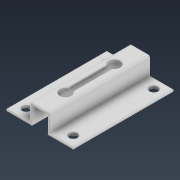
# Autodesk Inventor part: part1pasador
Saved by Autodesk Inventor 2021.2 (Build 252289000, 289)
## iProperties
Created: 2026-09-01
Part Number: part1pasador
Material: Generic
Document SubType Name: Modeling
Designer: Tecnica
Density: 1 g/cm^3
Appearance: Default
Author: Tecnica
Autodesk Inventor part; units mm, degrees
ref_plane "YZ Plane" through (0, 0, 0) normal (1, 0, 0) x (0, 1, 0)
ref_plane "XZ Plane" through (0, 0, 0) normal (0, 1, 0) x (-1, 0, 0)
ref_plane "XY Plane" through (0, 0, 0) normal (0, 0, 1) x (1, 0, 0)
sketch "Sketch1" plane through (0, 0, 0) normal (0, 1, 0) x (-1, 0, 0)
  line L0 (-20, 30) -> (20, 30)
  line L1 (20, 30) -> (20, -30)
  line L2 (20, -30) -> (-20, -30)
  line L3 (-20, -30) -> (-20, 30)
  line L4 (-20, 30) -> (20, -30) construction
  line L5 (20, 30) -> (-20, -30) construction
  point P0 (0, 0)
  dimension "d0" = 40
  dimension "d1" = 60
  constraints: 12 end point, 2 midpoint, 2 parallel, 1 horizontal, 1 perpendicular
  measures "d0" distance of L1.end L2.end
  measures "d1" distance of L0.end L1.end
extrude "Extrusion1" add sketch "Sketch1" along normal blind 12
sketch "Sketch2" plane through (-20, 0, 30) normal (0, 0, 1) x (1, 0, 0)
  line L0 (0, 0) -> (0, 12) projected
  line L1 (0, 0) -> (0, 1.45)
  line L2 (0, 1.45) -> (14, 1.45)
  line L3 (14, 1.45) -> (14, 12)
  line L4 (40, 12) -> (0, 12) projected
  line L5 (14, 12) -> (26, 12)
  line L6 (26, 12) -> (26, 1.45)
  line L7 (26, 1.45) -> (40, 1.45)
  line L8 (40, 0) -> (40, 12) projected
  line L9 (0, 12) -> (14, 12)
  line L10 (14, 12) -> (14, 1.45)
  line L11 (14, 1.45) -> (0, 1.45)
  line L12 (0, 1.45) -> (0, 12)
  line L13 (26, 1.45) -> (40, 1.45)
  line L14 (40, 1.45) -> (40, 12)
  line L15 (40, 12) -> (26, 12)
  line L16 (26, 12) -> (26, 1.45)
  line L17 (14, 1.45) -> (15.45, 1.45)
  line L18 (15.45, 1.45) -> (15.45, 12)
  line L19 (14, 12) -> (14, 10.55)
  line L20 (14, 10.55) -> (26, 10.55)
  line L21 (26, 12) -> (24.55, 12)
  line L22 (24.55, 12) -> (24.55, 1.45)
  line L23 (15.45, 10.55) -> (24.55, 10.55)
  line L24 (24.55, 10.55) -> (24.55, 0)
  line L25 (24.55, 0) -> (15.45, 0)
  line L26 (15.45, 0) -> (15.45, 10.55)
  point P0 (20, 0)
  point P1 (24.55, 1.45)
  point P2 (24.55, 10.55)
  point P3 (15.45, 1.45)
  dimension "d4" = 1.45
  dimension "d5" = 14
  dimension "d6" = 12
  dimension "d10" = 1.45
  dimension "d11" = 1.45
  dimension "d12" = 1.45
  constraints: 48 end point, 12 point on line, 10 perpendicular, 6 parallel, 4 horizontal
  measures "d4" distance of L0.start L1.end
  measures "d5" distance of L1.end L2.end
  measures "d6" distance of L3.end L5.end
  measures "d10" distance of L2.end L17.end
  measures "d11" distance of L9.end L19.end
  measures "d12" distance of L15.end L21.end
extrude "Extrusion2" cut sketch "Sketch2" against normal up to surface (60 mm away) contours L0 L4 L3 L2 | L18 L20 L22 L24 L25 L26 | L4 L8 L7 L6
fillet "Fillet1" radius 0.5 6 edges at (-20, 1.45, 0) (20, 1.45, 0) (-20, 0, 0) (20, 0, 0) (-4.55, 0, 0) (4.55, 0, 0)
fillet "Fillet1" radius 0.6 2 edges at (4.55, 10.55, 0) (-4.55, 10.55, 0)
fillet "Fillet1" radius 1.1 2 edges at (6, 12, 0) (-6, 12, 0)
sketch "Sketch3" plane through (-6, 1.45, 30) normal (0, 1, 0) x (1, 0, 0)
  line L0 (-14, 60) -> (-14, 0) projected
  line L1 (26, 0) -> (26, 60) projected
  line L2 (-14, 60) -> (26, 60)
  line L3 (26, 60) -> (26, 0)
  line L4 (26, 0) -> (-14, 0)
  line L5 (-14, 0) -> (-14, 60)
  line L6 (-14, 60) -> (-8, 60)
  line L7 (-8, 60) -> (-8, 54)
  line L8 (-8, 54) -> (-14, 54)
  line L9 (-14, 54) -> (-14, 60)
  circle A0 centre (-8, 54) radius 2.5
  line L10 (26, 60) -> (20, 60)
  line L11 (20, 60) -> (20, 54)
  line L12 (20, 54) -> (26, 54)
  line L13 (26, 54) -> (26, 60)
  circle A1 centre (20, 54) radius 2.5
  line L14 (26, 0) -> (25.5, 0) projected
  line L15 (26, 0) -> (20, 0)
  line L16 (20, 0) -> (20, 6)
  line L17 (20, 6) -> (26, 6)
  line L18 (26, 6) -> (26, 0)
  line L19 (-14, 0) -> (-8, 0)
  line L20 (-8, 0) -> (-8, 6)
  line L21 (-8, 6) -> (-14, 6)
  line L22 (-14, 6) -> (-14, 0)
  circle A2 centre (-8, 6) radius 2.5
  circle A3 centre (20, 6) radius 2.5
  point P0 (6, 30)
  dimension "d15" = 6
  dimension "d16" = 6
  dimension "d17" = 5
  dimension "d18" = 6
  dimension "d19" = 6
  dimension "d20" = 5
  dimension "d21" = 6
  dimension "d22" = 6
  dimension "d23" = 5
  dimension "d24" = 5
  dimension "d25" = 6
  dimension "d26" = 6
  constraints: 40 end point, 10 parallel, 5 horizontal, 5 perpendicular, 4 centre point, 4 coincident
  measures "d15" distance of L7.end L8.end
  measures "d16" distance of L6.end L7.end
  measures "d17" diameter of A0
  measures "d18" distance of L11.end L12.end
  measures "d19" distance of L10.end L11.end
  measures "d20" diameter of A1
  measures "d21" distance of L20.end L21.end
  measures "d22" distance of L19.end L20.end
  measures "d23" diameter of A2
  measures "d24" diameter of A3
  measures "d25" distance of L16.end L17.end
  measures "d26" distance of L15.end L16.end
extrude "Extrusion3" cut sketch "Sketch3" against normal blind 12 contours A0 L7 L8 | L8 L7 A0 | A2 L20 L21 | L21 L20 A2 | A1 L12 L11 | L11 L12 A1 | A3 L17 L16 | L16 L17 A3
sketch "Sketch4" plane through (0, 12, 0) normal (0, 1, 0) x (1, 0, 0)
  line L0 (3.95, 30) -> (-3.95, 30) projected
  line L1 (0, 30) -> (0, 18)
  line L2 (-3.95, -30) -> (3.95, -30) projected
  line L3 (0, -30) -> (0, -18)
  line L4 (0, 18) -> (0, 14.575)
  line L5 (0, -18) -> (0, -14.575)
  circle A0 centre (0, 14.575) radius 3.425
  circle A1 centre (0, -14.575) radius 3.425
  line L6 (0, 14.575) -> (1.7125, 14.575)
  line L7 (1.7125, 14.575) -> (1.7125, -14.575)
  line L8 (1.7125, -14.575) -> (0, -14.575)
  line L9 (0, -14.575) -> (0, 14.575)
  line L10 (0, 14.575) -> (1.7125, 14.575) construction
  line L11 (0, -14.575) -> (-1.7125, -14.575)
  line L12 (-1.7125, -14.575) -> (-1.7125, 14.575)
  line L13 (-1.7125, 14.575) -> (0, 14.575)
  line L14 (0, 14.575) -> (0, -14.575)
  point P0 (0, 0)
  point P1 (1.7125, -11.6089)
  point P2 (1.7125, 11.6089)
  point P3 (-1.7125, 11.6089)
  point P4 (-1.7125, -11.6089)
  dimension "d29" = 12
  dimension "d30" = 12
  dimension "d31" = 3.425
  dimension "d32" = 3.425
  dimension "d33" = 1.7125
  dimension "d34" = 0
  dimension "d35" = 1.7125
  constraints: 26 end point, 4 parallel, 4 vertical, 2 coincident, 2 horizontal, 2 midpoint, 2 perpendicular, 1 collinear, 1 point on line, 6 other
  measures "d29" distance of L1.start L1.end
  measures "d30" distance of L3.start L3.end
  measures "d31" distance of L1.end L4.end
  measures "d32" distance of L3.end L5.end
  measures "d33" distance of L6.start L6.end
  measures "d34" distance between parallel lines of L6 L10
  measures "d35" distance of L8.end L11.end
extrude "Extrusion4" cut sketch "Sketch4" against normal blind 12
fillet "Fillet2" radius 0.5 44 edges at (19.8536, 1.3036, 30) (20, 0.725, 30) (19.8536, 0.1464, 30) (12.275, 0, 30) (4.6964, 0.1464, 30) (4.55, 5.225, 30) (4.3743, 10.3743, 30) (0, 10.55, 30) (-4.3743, 10.3743, 30) (-4.55, 5.225, 30) (-4.6964, 0.1464, 30) (-12.275, 0, 30) (-19.8536, 0.1464, 30) (-20, 0.725, 30) (-19.8536, 1.3036, 30) (-12.75, 1.45, 30) (12.75, 1.45, 30) (5.6778, 11.6778, 30) (0, 12, 30) (-5.6778, 11.6778, 30) (-6, 6.175, 30) (6, 6.175, 30) (19.8536, 1.3036, -30) (20, 0.725, -30) (19.8536, 0.1464, -30) (12.275, 0, -30) (4.6964, 0.1464, -30) (4.55, 5.225, -30) (4.3743, 10.3743, -30) (0, 10.55, -30) (-4.3743, 10.3743, -30) (-4.55, 5.225, -30) (-4.6964, 0.1464, -30) (-12.275, 0, -30) (-19.8536, 0.1464, -30) (-20, 0.725, -30) (-19.8536, 1.3036, -30) (-12.75, 1.45, -30) (12.75, 1.45, -30) (5.6778, 11.6778, -30) (0, 12, -30) (-5.6778, 11.6778, -30) (-6, 6.175, -30) (6, 6.175, -30)
equation "\"d10\" = d4"
equation "\"d11\" = d4"
equation "\"d12\" = d4"
equation "\"d18\" = d15"
equation "\"d19\" = d16"
equation "\"d20\" = d17"
equation "\"d21\" = d15"
equation "\"d22\" = d16"
equation "\"d23\" = d17"
equation "\"d24\" = d17"
equation "\"d25\" = d15"
equation "\"d26\" = d16"
equation "\"d30\" = d29"
equation "\"d32\" = d31"
body "Solid1"
